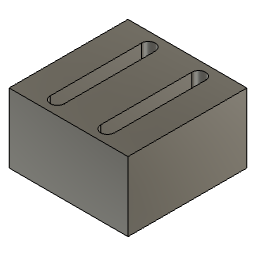
wheel_spacer_c2 v1 (Autodesk Fusion 360 design; units mm, degrees)
Autodesk Fusion 360 part; units mm, degrees
sketch "Sketch1" plane through (0, 0, 0) normal (0, 0, 1) x (1, 0, 0)
  line L0 (0, 0) -> (60, 0)
  line L1 (60, 0) -> (60, 60)
  line L2 (60, 60) -> (0, 60)
  line L3 (0, 60) -> (0, 0)
  line L4 (60, 60) -> (0, 0) construction
  line L5 (0, 60) -> (60, 0) construction
  line L6 (30, 30) -> (30, 60) construction
  line L7 (30, 30) -> (30, 0) construction
  line L8 (17.3, 60) -> (17.3, 0) construction
  line L9 (42.7, 60) -> (42.7, 0) construction
  line L10 (0, 7) -> (60, 7) construction
  line L11 (0, 53) -> (60, 53) construction
  circle A0 centre (17.3, 53) radius 3.5
  circle A1 centre (17.3, 7) radius 3.5
  circle A2 centre (42.7, 7) radius 3.5
  circle A3 centre (42.7, 53) radius 3.5
  line L12 (13.8, 53) -> (13.8, 7)
  line L13 (20.8, 7) -> (20.8, 53)
  line L14 (39.2, 53) -> (39.2, 7)
  line L15 (46.2, 7) -> (46.2, 53)
  dimension "d1" = 60
  dimension "d2" = 60
  dimension "d3" = 12.7
  dimension "d4" = 12.7
  dimension "d5" = 23
  dimension "d8" = 23
  dimension "d9" = 7
  dimension "d10" = 7
  dimension "d11" = 7
  dimension "d12" = 7
  constraint horizontal L0
  constraint vertical L1
  constraint horizontal L2
  constraint vertical L3
  constraint coincident L0.start L3.end
  constraint midpoint L4 L6.start
  constraint midpoint L2 L6.end
  constraint midpoint L0 L7.end
  constraint coincident L2 L8.start
  constraint coincident L0 L8.end
  constraint perpendicular L0 L8
  constraint coincident L2 L9.start
  constraint coincident L0 L9.end
  constraint perpendicular L0 L9
  constraint coincident L3 L10.start
  constraint coincident L1 L10.end
  constraint perpendicular L1 L10
  constraint coincident L3 L11.start
  constraint coincident L1 L11.end
  constraint perpendicular L1 L11
  constraint coincident L8 A0.centre
  constraint coincident L11 A0.centre
  constraint coincident L8 A1.centre
  constraint coincident L10 A1.centre
  constraint coincident L10 A2.centre
  constraint coincident L9 A2.centre
  constraint coincident L11 A3.centre
  constraint coincident L9 A3.centre
  constraint coincident L11 L12.start
  constraint coincident A0 L12.start
  constraint coincident A1 L12.end
  constraint coincident L10 L12.end
  constraint coincident A1 L13.start
  constraint coincident L10 L13.start
  constraint coincident L11 L13.end
  constraint coincident A0 L13.end
  constraint coincident L11 L14.start
  constraint coincident A3 L14.start
  constraint coincident A2 L14.end
  constraint coincident L10 L14.end
  constraint coincident A2 L15.start
  constraint coincident L10 L15.start
  constraint coincident A3 L15.end
  constraint coincident L11 L15.end
  measures "d1" distance of L0.start L0.end
  measures "d2" distance of L0.start L2.end
  measures "d3" distance of L6 L8
  measures "d4" distance of L6 L9
  measures "d5" distance of L6.start L10
  measures "d8" distance of L6.start L11
  measures "d9" diameter of A0
  measures "d10" diameter of A1
  measures "d11" diameter of A2
  measures "d12" diameter of A3
extrude "Extrude1" add sketch "Sketch1" along normal blind 35
